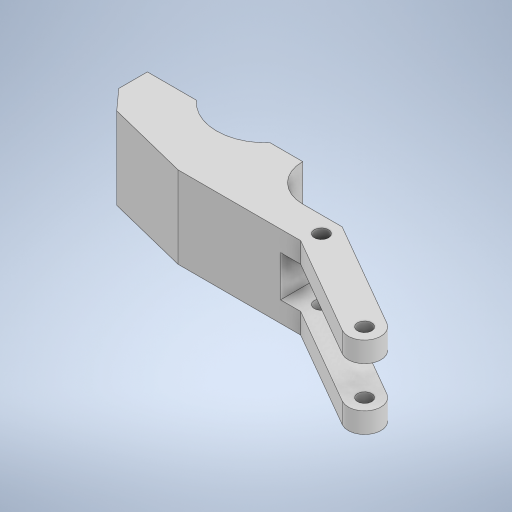
# Autodesk Inventor part: Gripper
Saved by Autodesk Inventor 2023 (Build 270158000, 158)
## iProperties
Created: 2024-07-18
Part Number: Gripper
Material: Generic
Document SubType Name: Modeling
Designer: Swoby
Density: 1 g/cm^3
Appearance: Default
Author: Swoby
Autodesk Inventor part; units mm, degrees
ref_plane "YZ Plane" through (0, 0, 0) normal (1, 0, 0) x (0, 1, 0)
ref_plane "XZ Plane" through (0, 0, 0) normal (0, 1, 0) x (-1, 0, 0)
ref_plane "XY Plane" through (0, 0, 0) normal (0, 0, 1) x (1, 0, 0)
sketch "Sketch1" plane through (0, 0, 0) normal (0, 1, 0) x (-1, 0, 0)
  arc A0 (10, -13) -> (1, -4) centre (1, -13) ccw
  line L0 (10, -13) -> (18, -13)
  arc A1 (36, -13) -> (18, -13) centre (27, -20.9373) ccw
  line L1 (36, -13) -> (48, -13)
  line L2 (23.5, 4) -> (43.5, -1)
  line L3 (43.5, -1) -> (48, -6)
  line L4 (48, -6) -> (48, -13)
  circle A2 centre (-7.5718, 0) radius 1.75
  circle A3 centre (-32.5718, 14.4338) radius 1.75
  line L5 (-32.5718, 14.4338) -> (-7.5718, 0) construction
  line L6 (-7.5718, 0) -> (0, 0) construction
  line L7 (-34.5718, 10.9697) -> (-8.6436, -4)
  arc A4 (-30.5718, 17.8979) -> (-34.5718, 10.9697) centre (-32.5718, 14.4338) ccw
  line L8 (1, -4) -> (-8.6436, -4)
  line L9 (-30.5718, 17.8979) -> (-6.5, 4)
  line L10 (-6.5, 4) -> (23.5, 4)
  point P0 (-21.6077, 3.4848)
  point P1 (-20.0718, 7.2169)
  dimension "d3" = 1
  dimension "d8" = 12
  dimension "d9" = 8
  dimension "d10" = 18
  dimension "d11" = 9
  dimension "d12" = 9
  dimension "d13" = 12
  dimension "d24" = 3.5
  dimension "d25" = 3.5
  dimension "d26" = 150
  dimension "d36" = 4
  dimension "d38" = 9
  dimension "d40" = 4
  dimension "d41" = 25
  dimension "d54" = 4
  dimension "d55" = 4
  dimension "d56" = 7
  dimension "d57" = 30
  dimension "d58" = 20
  dimension "d59" = 4.5
  dimension "d60" = 5
  dimension "d61" = 5
  constraints: 22 end point, 6 point on circle, 5 centre point, 3 horizontal, 3 parallel, 2 midpoint, 1 coincident, 1 collinear, 1 vertical
  measures "d3" horizontal distance of L6.end L8.start
  measures "d8" distance of L1.start L1.end
  measures "d9" distance of L0.start L0.end
  measures "d10" distance of L0.end L1.start
  measures "d11" horizontal distance of L8.start L0.start
  measures "d12" horizontal distance of L8.start L0.start
  measures "d13" radius of A1
  measures "d24" diameter of A2
  measures "d25" diameter of A3
  measures "d26" angle of L5 L6
  measures "d36" distance between parallel lines of L8 L6
  measures "d38" radius of A0
  measures "d40" radius of A4
  measures "d41" horizontal distance of L5.start L5.end
  measures "d54" distance between parallel lines of L5 L9
  measures "d55" distance between parallel lines of L7 L5
  measures "d56" distance of L3.end L1.end
  measures "d57" distance of L9.end L2.start
  measures "d58" horizontal distance of L2.start L2.end
  measures "d59" horizontal distance of L2.end L3.end
  measures "d60" vertical distance of L3.end L2.end
  measures "d61" vertical distance of L2.end L2.start
extrude "Extrusion1" add sketch "Sketch1" along normal blind 20 contours A0 L8 L7 A4 L9 L10 L2 L3 L4 L1 A1 L0 | A2 | A3
sketch "Sketch2" plane through (8.6436, 0, -4) normal (0, 0, -1) x (-1, 0, 0)
  line L0 (-27.9282, 0) -> (-27.9282, 20) projected
  line L1 (-27.9282, 15) -> (7.0718, 15)
  line L2 (7.0718, 15) -> (7.0718, 5)
  line L3 (7.0718, 5) -> (-27.9282, 5)
  line L4 (-27.9282, 5) -> (-27.9282, 15)
  line L5 (-25.9282, 20) -> (0, 20) projected
  line L6 (-25.9282, 0) -> (0, 0) projected
  point P0 (8.6436, 0)
  dimension "d47" = 5
  dimension "d48" = 5
  dimension "d49" = 35
  constraints: 8 end point, 2 parallel, 1 horizontal, 1 perpendicular, 1 point on line
  measures "d47" distance between parallel lines of L1 L5
  measures "d48" distance between parallel lines of L6 L3
  measures "d49" distance of L1.start L1.end
extrude "Extrusion2" cut sketch "Sketch2" against normal through all
extrude "Extrusion3" cut sketch "Sketch1" along normal through all contours A2 | A3
body "Solid1"
